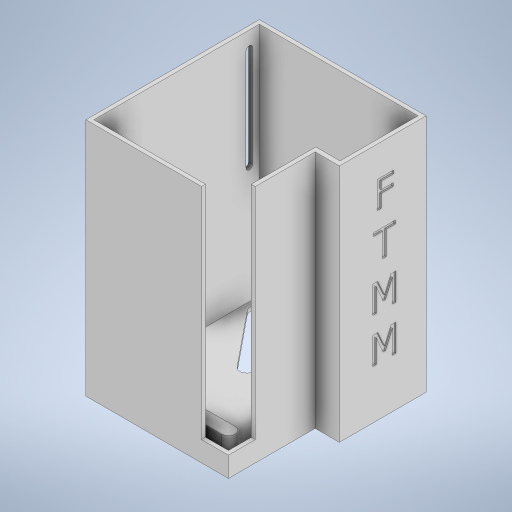
# Autodesk Inventor part: cover windshield
Saved by Autodesk Inventor 2023 (Build 270158030, 158C)
## iProperties
Created: 2023-03-05
Part Number: cover windshield
Material: Generic
Document SubType Name: Modeling
Designer: fatih
Density: 1 g/cm^3
Appearance: Default
Author: fatih
Autodesk Inventor part; units mm, degrees
ref_plane "YZ Plane" through (0, 0, 0) normal (1, 0, 0) x (0, 1, 0)
ref_plane "XZ Plane" through (0, 0, 0) normal (0, 1, 0) x (-1, 0, 0)
ref_plane "XY Plane" through (0, 0, 0) normal (0, 0, 1) x (1, 0, 0)
sketch "Sketch1" plane through (0, 0, 0) normal (0, 1, 0) x (-1, 0, 0)
  line L0 (0, 0) -> (100, 0)
  line L1 (100, 0) -> (100, -123)
  line L2 (100, -123) -> (0, -123)
  line L3 (0, -123) -> (0, 0)
  dimension "d0" = 123
  dimension "d1" = 100
  constraints: 8 end point, 2 parallel, 1 horizontal, 1 perpendicular
  measures "d0" distance of L0.end L1.end
  measures "d1" distance of L0.start L0.end
extrude "Extrusion1" add sketch "Sketch1" along normal blind 175
shell "Shell1" thickness 3 outward yes removed faces 1 at (-33.3333, 175, -41)
sketch "Sketch3" plane through (-103, -3, -126) normal (-1, 0, 0) x (0, 0, 1)
  line L0 (129, 0) -> (0, 0) projected
  line L1 (3, 178) -> (126, 178) projected
  line L2 (0, 0) -> (20, 0)
  line L3 (20, 0) -> (20, 178)
  line L4 (20, 178) -> (0, 178)
  line L5 (0, 178) -> (0, 0)
  line L6 (0, 0) -> (0, 15)
  line L7 (0, 0) -> (0, 178) projected
  line L8 (0, 15) -> (20, 15)
  point P0 (126, 3)
  point P1 (3, 178)
  dimension "d7" = 15
  dimension "d10" = 20
  constraints: 12 end point, 3 point on line, 2 parallel, 2 perpendicular, 1 horizontal
  measures "d7" distance of L0.end L6.end
  measures "d10" distance of L6.end L8.end
extrude "Extrusion3" cut sketch "Sketch3" against normal blind 20 contours L8 L5 L4 L1 L3
sketch "Sketch6" plane through (-100, 0, -123) normal (0, 1, 0) x (1, 0, 0)
  line L0 (100, 0) -> (0, 0) projected
  line L1 (85, -15) -> (15, -15) construction
  line L2 (85, -10) -> (15, -10)
  line L3 (15, -20) -> (85, -20)
  arc A0 (85, -20) -> (85, -10) centre (85, -15) ccw
  arc A1 (15, -10) -> (15, -20) centre (15, -15) ccw
  point P0 (100, -123)
  point P1 (50, 0)
  point P2 (50, -10)
  dimension "d20" = 70
  dimension "d21" = 10
  constraints: 8 end point, 4 point on circle, 4 tangent, 2 centre point, 2 midpoint, 1 parallel
  measures "d20" distance of L2.start L2.end
  measures "d21" distance of point (50, 0) point (50, -10)
extrude "Extrusion5" add sketch "Sketch6" along normal blind 10
sketch "Sketch7" plane through (-103, -3, -126) normal (-1, 0, 0) x (0, 0, 1)
  line L0 (0, 0) -> (0, 178) projected
  line L1 (129, 0) -> (129, 178) projected
  line L2 (0, 0) -> (129, 0) projected
  line L3 (129, 178) -> (64.5, 178)
  line L4 (64.5, 178) -> (64.5, 0)
  line L5 (64.5, 0) -> (129, 0)
  line L6 (129, 0) -> (129, 178)
  point P0 (126, 3)
  constraints: 8 end point, 2 parallel, 1 horizontal, 1 midpoint, 1 perpendicular
extrude "Extrusion6" add sketch "Sketch7" along normal blind 18
sketch "Sketch8" plane through (-100, 0, 0) normal (1, 0, 0) x (0, 0, -1)
  line L0 (123, 0) -> (0, 0) projected
  line L1 (-3, 175) -> (126, 175) projected
  line L2 (0, 0) -> (58, 0)
  line L3 (58, 0) -> (58, 175)
  line L4 (58, 175) -> (0, 175)
  line L5 (0, 175) -> (0, 0)
  dimension "d27" = 58
  constraints: 8 end point, 2 parallel, 1 horizontal, 1 perpendicular, 1 point on line
  measures "d27" distance of L4.end L3.end
extrude "Extrusion7" cut sketch "Sketch8" against normal blind 18
sketch "Sketch9" plane through (0, -3, 0) normal (0, -1, 0) x (1, 0, 0)
  line L0 (0, 0) -> (0, -123) projected
  line L1 (0, -61.5) -> (-100, -61.5)
  line L2 (-100, -123) -> (-100, -58) projected
  line L3 (-100, -61.5) -> (-100, 0)
  line L4 (-50, -61.5) -> (-50, 0)
  line L5 (-8.5984, -10.5761) -> (-41.4016, -50.9239) construction
  line L6 (-12.478, -7.4219) -> (-45.2812, -47.7698)
  line L7 (-37.522, -54.0781) -> (-4.7188, -13.7302)
  arc A0 (-4.7188, -13.7302) -> (-12.478, -7.4219) centre (-8.5984, -10.5761) ccw
  arc A1 (-45.2812, -47.7698) -> (-37.522, -54.0781) centre (-41.4016, -50.9239) ccw
  line L8 (-58.5984, -10.5761) -> (-91.4016, -50.9239) construction
  line L9 (-62.478, -7.4219) -> (-95.2812, -47.7698)
  line L10 (-87.522, -54.0781) -> (-54.7188, -13.7302)
  arc A2 (-54.7188, -13.7302) -> (-62.478, -7.4219) centre (-58.5984, -10.5761) ccw
  arc A3 (-95.2812, -47.7698) -> (-87.522, -54.0781) centre (-91.4016, -50.9239) ccw
  point P0 (-25, -30.75)
  point P1 (-75, -30.75)
  dimension "d30" = 26
  dimension "d31" = 10
  dimension "d32" = 26
  dimension "d33" = 10
  constraints: 22 end point, 8 point on circle, 8 tangent, 4 centre point, 4 midpoint, 2 parallel, 2 vertical, 1 horizontal, 1 point on line
  measures "d30" distance of point (-25, -30.75) L5.end
  measures "d31" diameter of A1
  measures "d32" distance of point (-75, -30.75) L8.end
  measures "d33" diameter of A3
extrude "Extrusion8" cut sketch "Sketch9" against normal blind 18
sketch "Sketch10" plane through (3, -3, 3) normal (1, 0, 0) x (0, 0, -1)
  line L0 (3, 3) -> (3, 178) projected
  line L1 (3, 90.5) -> (8, 90.5)
  line L2 (8, 90.5) -> (8, 165.5)
  line L3 (0, 178) -> (64.5, 178) projected
  line L4 (8, 165.5) -> (13, 165.5)
  line L5 (13, 165.5) -> (13, 90.5)
  line L6 (13, 90.5) -> (8, 90.5)
  line L7 (10.5, 128) -> (13, 128)
  line L8 (10.5, 90.5) -> (10.5, 165.5) construction
  line L9 (8, 90.5) -> (8, 165.5)
  line L10 (13, 165.5) -> (13, 90.5)
  arc A0 (8, 90.5) -> (13, 90.5) centre (10.5, 90.5) ccw
  arc A1 (13, 165.5) -> (8, 165.5) centre (10.5, 165.5) ccw
  point P0 (13, 90.5)
  point P1 (13, 165.5)
  dimension "d36" = 5
  dimension "d37" = 75
  dimension "d38" = 5
  constraints: 20 end point, 4 midpoint, 4 perpendicular, 4 point on circle, 4 tangent, 2 centre point, 1 horizontal, 1 parallel, 1 point on line
  measures "d36" distance of L1.start L1.end
  measures "d37" distance of L1.end L2.end
  measures "d38" distance of L2.end L4.end
extrude "Extrusion9" cut sketch "Sketch10" against normal blind 18
sketch "Sketch11" plane through (-121, -3, -126) normal (-1, 0, 0) x (0, 0, 1)
  line L0 (87.3766, 155.2155) -> (108.576, 155.2155) construction
  line L1 (108.576, 155.2155) -> (108.576, 36.4271) construction
  line L2 (108.576, 36.4271) -> (87.3766, 36.4271) construction
  line L3 (87.3766, 36.4271) -> (87.3766, 155.2155) construction
  line L4 (104.7916, 152.8492) -> (95.4885, 152.8492)
  line L5 (95.4885, 152.8492) -> (95.4885, 147.209)
  line L6 (95.4885, 147.209) -> (104.4026, 147.209)
  line L7 (104.4026, 147.209) -> (104.4026, 144.8427)
  line L8 (104.4026, 144.8427) -> (95.4885, 144.8427)
  line L9 (95.4885, 144.8427) -> (95.4885, 135.2155)
  line L10 (95.4885, 135.2155) -> (92.8305, 135.2155)
  line L11 (92.8305, 135.2155) -> (92.8305, 155.2155)
  line L12 (92.8305, 155.2155) -> (104.7916, 155.2155)
  line L13 (104.7916, 155.2155) -> (104.7916, 152.8492)
  line L14 (96.6311, 102.286) -> (96.6311, 119.9197)
  line L15 (96.6311, 119.9197) -> (89.9212, 119.9197)
  line L16 (89.9212, 119.9197) -> (89.9212, 122.286)
  line L17 (89.9212, 122.286) -> (105.999, 122.286)
  line L18 (105.999, 122.286) -> (105.999, 119.9197)
  line L19 (105.999, 119.9197) -> (99.2891, 119.9197)
  line L20 (99.2891, 119.9197) -> (99.2891, 102.286)
  line L21 (99.2891, 102.286) -> (96.6311, 102.286)
  line L22 (106.5501, 69.3566) -> (103.892, 69.3566)
  line L23 (103.892, 69.3566) -> (103.892, 86.5851)
  line L24 (103.892, 86.5851) -> (98.6732, 74.8671)
  line L25 (98.6732, 74.8671) -> (97.0525, 74.8671)
  line L26 (97.0525, 74.8671) -> (91.8823, 86.5851)
  line L27 (91.8823, 86.5851) -> (91.8823, 69.3566)
  line L28 (91.8823, 69.3566) -> (89.4026, 69.3566)
  line L29 (89.4026, 69.3566) -> (89.4026, 89.3566)
  line L30 (89.4026, 89.3566) -> (93.033, 89.3566)
  line L31 (93.033, 89.3566) -> (98.0249, 78.222)
  line L32 (98.0249, 78.222) -> (102.8548, 89.3566)
  line L33 (102.8548, 89.3566) -> (106.5501, 89.3566)
  line L34 (106.5501, 89.3566) -> (106.5501, 69.3566)
  line L35 (106.5501, 36.4271) -> (103.892, 36.4271)
  line L36 (103.892, 36.4271) -> (103.892, 53.6556)
  line L37 (103.892, 53.6556) -> (98.6732, 41.9376)
  line L38 (98.6732, 41.9376) -> (97.0525, 41.9376)
  line L39 (97.0525, 41.9376) -> (91.8823, 53.6556)
  line L40 (91.8823, 53.6556) -> (91.8823, 36.4271)
  line L41 (91.8823, 36.4271) -> (89.4026, 36.4271)
  line L42 (89.4026, 36.4271) -> (89.4026, 56.4271)
  line L43 (89.4026, 56.4271) -> (93.033, 56.4271)
  line L44 (93.033, 56.4271) -> (98.0249, 45.2926)
  line L45 (98.0249, 45.2926) -> (102.8548, 56.4271)
  line L46 (102.8548, 56.4271) -> (106.5501, 56.4271)
  line L47 (106.5501, 56.4271) -> (106.5501, 36.4271)
  point P0 (126, 3)
  constraints: 2 other
emboss "Emboss1" sketch "Sketch11" operation cut depth 1 direction (1, 0, 0)
body "Solid1"
